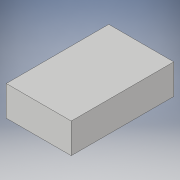
# Autodesk Inventor part: Battery Charger Repreentation
Saved by Autodesk Inventor 2018 (Build 220112000, 112)
## iProperties
Created: 2018-12-11
Part Number: Battery Charger Repreentation
Material: Generic
Document SubType Name: Modeling
Designer: Gabriel
Density: 1 g/cm^3
Appearance: Default
Author: Gabriel
Autodesk Inventor part; units mm, degrees
ref_plane "YZ Plane" through (0, 0, 0) normal (1, 0, 0) x (0, 1, 0)
ref_plane "XZ Plane" through (0, 0, 0) normal (0, 1, 0) x (-1, 0, 0)
ref_plane "XY Plane" through (0, 0, 0) normal (0, 0, 1) x (1, 0, 0)
sketch "Sketch1" plane through (0, 0, 0) normal (0, 1, 0) x (-1, 0, 0)
  line L0 (6.7464, 15.2068) -> (-158.3536, 15.2068)
  line L1 (-158.3536, 15.2068) -> (-158.3536, -245.1432)
  line L2 (-158.3536, -245.1432) -> (6.7464, -245.1432)
  line L3 (6.7464, -245.1432) -> (6.7464, 15.2068)
  point P0 (0, 0)
  dimension "d0" = 165.1
  dimension "d1" = 260.35
  constraints: 8 end point, 2 parallel, 1 horizontal, 1 perpendicular
  measures "d0" distance of L2.end L1.end
  measures "d1" distance of L1.end L0.end
extrude "Extrusion1" add sketch "Sketch1" along normal blind 76.2
body "Solid1"
